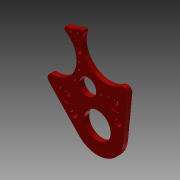
# Autodesk Inventor part: OutlineSketch1
Saved by Autodesk Inventor 2013 (Build 170138000, 138)
## iProperties
Created: 2013-06-03
Part Number: OutlineSketch1
Material: Aluminum 6061
Document SubType Name: Modeling
Designer: mvarma
Density: 2.71 g/cm^3
Mass: 149.846 g
Surface Area: 274.597 cm^2
Volume: 55.2937 cm^3
Author: mvarma
Autodesk Inventor part; units mm, degrees
ref_plane "YZ Plane" through (0, 0, 0) normal (1, 0, 0) x (0, 1, 0)
ref_plane "XZ Plane" through (0, 0, 0) normal (0, 1, 0) x (-1, 0, 0)
ref_plane "XY Plane" through (0, 0, 0) normal (0, 0, 1) x (1, 0, 0)
sketch "Sketch1" plane through (0, 0, 0) normal (0, 0, 1) x (1, 0, 0)
  line L0 (0, 0) -> (304.8, 0) construction
  line L1 (304.8, 0) -> (304.8, 50.8) construction
  line L2 (304.8, 50.8) -> (0, 50.8) construction
  line L3 (0, 50.8) -> (0, 0) construction
  circle A0 centre (152.4, 23.8125) radius 17.4625
  arc A1 (186.5267, 20.4696) -> (127.7268, 0) centre (152.4, 23.8125) ccw
  circle A2 centre (152.4, 23.8125) radius 26.035 construction
  line L4 (152.4, 23.8125) -> (139.52, 61.741) construction
  circle A3 centre (139.52, 61.741) radius 9.525 construction
  circle A4 centre (139.52, 61.741) radius 17.78 construction
  circle A5 centre (91.5619, 85.09) radius 31.75 construction
  arc A6 (133.1868, 119.4006) -> (182.1011, 83.8499) centre (163.3424, 109.4657) ccw
  circle A7 centre (109.5312, 150.0506) radius 31.75 construction
  line L5 (0, 50.8) -> (0, 53.34) construction
  line L6 (0, 53.34) -> (304.8, 53.34) construction
  line L7 (304.8, 53.34) -> (304.8, 50.8) construction
  circle A8 centre (139.52, 61.741) radius 21.59 construction
  circle A9 centre (152.4, 23.8125) radius 46.99 construction
  circle A10 centre (152.4, 23.8125) radius 50.8 construction
  arc A11 (86.3865, 79.4564) -> (92.4363, 92.6899) centre (91.5619, 85.09) ccw construction
  circle A12 centre (163.3424, 109.4657) radius 7.65 construction
  arc A13 (116.7749, 152.5104) -> (102.2875, 147.5907) centre (109.5312, 150.0506) ccw construction
  circle A14 centre (139.52, 61.741) radius 22.9 construction
  line L8 (86.3865, 79.4564) -> (124.0276, 44.8769) construction
  line L9 (170.8782, 108.1486) -> (162.078, 57.7984) construction
  line L10 (92.4363, 92.6899) -> (91.5619, 85.09) construction
  line L11 (91.5619, 85.09) -> (86.3865, 79.4564) construction
  circle A15 centre (127.6738, 96.6252) radius 3.175 construction
  circle A16 centre (127.6738, 96.6252) radius 7.9375 construction
  line L12 (92.4363, 92.6899) -> (126.7664, 88.7398) construction
  line L13 (133.1953, 90.9229) -> (158.0208, 114.9615) construction
  line L14 (158.0208, 114.9615) -> (163.3424, 109.4657) construction
  line L15 (170.8782, 108.1486) -> (163.3424, 109.4657) construction
  line L16 (139.52, 61.741) -> (127.6738, 96.6252) construction
  line L17 (91.5619, 85.09) -> (163.3424, 109.4657) construction
  line L18 (152.4, 23.8125) -> (91.5619, 85.09) construction
  line L19 (152.4, 23.8125) -> (163.3424, 109.4657) construction
  circle A17 centre (127.6738, 96.6252) radius 9.2075 construction
  circle A18 centre (127.6738, 96.6252) radius 6.1595 construction
  arc A19 (92.4363, 92.6899) -> (86.3865, 79.4564) centre (91.5619, 85.09) ccw construction
  circle A20 centre (163.3424, 109.4657) radius 25.4 construction
  circle A21 centre (109.5312, 150.0506) radius 25.4 construction
  line L20 (104.7627, 113.9656) -> (78.361, 56.2144) construction
  circle A22 centre (91.5619, 85.09) radius 25.4 construction
  line L21 (139.595, 160.2598) -> (79.4674, 139.8413) construction
  circle A23 centre (139.52, 61.741) radius 11.1125
  arc A24 (100.1373, 146.0575) -> (119.6802, 151.6232) centre (109.9088, 148.8404) ccw construction
  line L22 (109.0937, 151.2404) -> (85.4802, 141.8832) construction
  line L23 (109.9088, 148.8404) -> (85.4802, 141.8832) construction
  line L24 (109.0937, 151.2404) -> (132.7073, 160.5977) construction
  line L25 (109.9088, 148.8404) -> (134.3374, 155.7976) construction
  arc A25 (134.9211, 161.475) -> (130.4935, 159.7205) centre (132.7073, 160.5977) ccw construction
  arc A26 (132.0472, 155.1453) -> (136.6276, 156.4498) centre (134.3374, 155.7976) ccw construction
  arc A27 (132.0472, 155.1453) -> (130.4935, 159.7205) centre (85.4802, 141.8832) ccw construction
  arc A28 (136.6276, 156.4498) -> (134.9211, 161.475) centre (85.4802, 141.8832) ccw construction
  line L26 (132.7073, 160.5977) -> (134.9211, 161.475) construction
  line L27 (134.3374, 155.7976) -> (136.6276, 156.4498) construction
  arc A29 (119.6802, 151.6232) -> (118.5392, 154.9834) centre (85.4802, 141.8832) ccw construction
  arc A30 (100.1373, 146.0575) -> (99.6483, 147.4975) centre (85.4802, 141.8832) ccw construction
  line L28 (104.4015, 107.0791) -> (92.7013, 84.5343) construction
  line L29 (81.0012, 61.9895) -> (90.3961, 85.5882) construction
  arc A31 (100.6718, 111.3992) -> (98.9102, 106.9744) centre (99.791, 109.1868) ccw construction
  arc A32 (103.3046, 104.9655) -> (105.4983, 109.1926) centre (104.4015, 107.0791) ccw construction
  arc A33 (103.3046, 104.9655) -> (98.9102, 106.9744) centre (81.0012, 61.9895) ccw construction
  line L30 (99.791, 109.1868) -> (100.6718, 111.3992) construction
  line L31 (104.4015, 107.0791) -> (105.4983, 109.1926) construction
  arc A34 (105.4983, 109.1926) -> (100.6718, 111.3992) centre (81.0012, 61.9895) ccw construction
  arc A35 (118.5392, 154.9834) -> (99.6483, 147.4975) centre (109.0937, 151.2404) ccw construction
  arc A36 (88.0213, 75.5164) -> (97.3814, 93.5522) centre (92.7013, 84.5343) ccw construction
  line L32 (90.3961, 85.5882) -> (99.791, 109.1868) construction
  line L33 (92.7013, 84.5343) -> (81.0012, 61.9895) construction
  arc A37 (88.0213, 75.5164) -> (86.6381, 76.1487) centre (81.0012, 61.9895) ccw construction
  arc A38 (97.3814, 93.5522) -> (94.1541, 95.0276) centre (81.0012, 61.9895) ccw construction
  arc A39 (94.1541, 95.0276) -> (86.6381, 76.1487) centre (90.3961, 85.5882) ccw construction
  line L34 (163.3424, 109.4657) -> (140.8985, 121.3583) construction
  line L35 (163.3424, 109.4657) -> (185.7862, 97.5731) construction
  circle A40 centre (139.52, 61.741) radius 22.9 construction
  arc A41 (102.2875, 147.5907) -> (116.7749, 152.5104) centre (109.5312, 150.0506) ccw construction
  arc A42 (102.2875, 147.5907) -> (102.6226, 146.7653) centre (109.5312, 150.0506) ccw construction
  circle A43 centre (90.3961, 85.5882) radius 31.75
  arc A44 (107.3265, 112.7153) -> (92.5282, 52.7848) centre (92.7013, 84.5343) ccw
  line L36 (100.6718, 111.3992) -> (102.1397, 115.0865) construction
  line L37 (105.4983, 109.1926) -> (107.3265, 112.7153) construction
  arc A45 (107.3265, 112.7153) -> (102.1397, 115.0865) centre (81.0012, 61.9895) ccw
  circle A46 centre (109.0937, 151.2404) radius 31.75
  arc A47 (120.148, 118.7867) -> (128.3292, 122.9801) centre (109.9088, 148.8404) ccw
  line L38 (134.9211, 161.475) -> (138.6107, 162.9371) construction
  line L39 (136.6276, 156.4498) -> (140.4445, 157.5369) construction
  arc A48 (140.4445, 157.5369) -> (138.6107, 162.9371) centre (85.4802, 141.8832) ccw
  line L40 (91.5619, 85.09) -> (109.5312, 150.0506) construction
  line L41 (109.5312, 150.0506) -> (163.3424, 109.4657) construction
  line L42 (139.52, 61.741) -> (109.5312, 150.0506) construction
  circle A49 centre (139.52, 61.741) radius 17.4625
  line L43 (139.52, 61.741) -> (122.0575, 61.741) construction
  line L44 (139.52, 61.741) -> (156.9825, 61.741) construction
  line L45 (139.52, 61.741) -> (156.9825, 61.741) construction
  circle A50 centre (139.52, 61.741) radius 26.71 construction
  circle A51 centre (111.304, 39.007) radius 9.525 construction
  circle A52 centre (175.745, 60.8903) radius 9.525 construction
  line L46 (0, 3.81) -> (304.8, 3.81) construction
  arc A53 (86.5066, 75.4886) -> (95.7233, 93.5981) centre (91.1149, 84.5434) ccw
  arc A54 (92.4843, 95.0479) -> (85.1185, 76.1099) centre (88.8014, 85.5789) ccw
  arc A55 (95.7233, 93.5981) -> (92.4843, 95.0479) centre (79.5941, 61.9064) ccw
  circle A56 centre (120.9278, 20.7284) radius 5.588
  circle A57 centre (179.6201, 39.9084) radius 5.588
  line L47 (152.4, 23.8125) -> (304.8, 25.4) construction
  line L48 (179.6201, 39.9084) -> (152.4, 23.8125) construction
  line L49 (152.4, 23.8125) -> (120.9278, 20.7284) construction
  line L50 (67.3436, 63.7559) -> (87.8831, 42.0684)
  line L51 (186.5267, 20.4696) -> (192.1727, 78.1076)
  arc A58 (109.8133, 111.2783) -> (111.3776, 117.1243) centre (111.5245, 113.9527) ccw
  arc A59 (128.3292, 122.9801) -> (133.1868, 119.4006) centre (130.1712, 120.3941) ccw
  arc A60 (111.3776, 117.1243) -> (120.148, 118.7867) centre (109.9088, 148.8404) ccw
  arc A61 (128.3292, 122.9801) -> (111.3776, 117.1243) centre (109.9088, 148.8404) ccw
  arc A62 (137.9937, 128.5839) -> (133.1868, 119.4006) centre (163.3424, 109.4657) ccw
  arc A63 (109.8133, 111.2783) -> (107.3265, 112.7153) centre (92.7013, 84.5343) ccw
  arc A64 (92.5282, 52.7848) -> (87.8831, 42.0684) centre (92.4936, 46.4349) ccw
  arc A65 (182.1011, 83.8499) -> (192.1727, 78.1076) centre (185.8529, 78.7267) ccw
  arc A66 (192.1727, 78.1076) -> (182.1011, 83.8499) centre (185.8529, 78.7267) ccw
  arc A67 (97.1053, 50.8) -> (92.5282, 52.7848) centre (92.4936, 46.4349) ccw
  arc A68 (87.8831, 42.0684) -> (97.1053, 50.8) centre (92.4936, 46.4349) ccw
  line L52 (87.8831, 42.0684) -> (127.5033, 0.2337)
  line L53 (192.1727, 78.1076) -> (194.9412, 106.3704)
  arc A69 (182.1011, 83.8499) -> (137.9937, 128.5839) centre (163.3424, 109.4657) ccw
  arc A70 (180.2515, 3.81) -> (186.5267, 20.4696) centre (152.4, 23.8125) ccw
  arc A71 (127.7268, 0) -> (180.2515, 3.81) centre (152.4, 23.8125) ccw
  arc A72 (92.5282, 52.7848) -> (109.8133, 111.2783) centre (92.7013, 84.5343) ccw
  arc A73 (133.1868, 119.4006) -> (128.3292, 122.9801) centre (130.1712, 120.3941) ccw
  arc A74 (111.3776, 117.1243) -> (109.8133, 111.2783) centre (111.5245, 113.9527) ccw
  point P0 (133.5823, 158.218)
  point P1 (102.1225, 108.1905)
  dimension "d122" = 63.5
  dimension "d1" = 50.8
  dimension "d2" = 34.925
  dimension "d3" = 23.8125
  dimension "d4" = 152.4
  dimension "d7" = 68.58
  dimension "d8" = 52.07
  dimension "d9" = 19.05
  dimension "d10" = 35.56
  dimension "d11" = 40.0558
  dimension "d12" = 63.5
  dimension "d13" = 63.5
  dimension "d14" = 63.5
  dimension "d15" = 2.54
  dimension "d16" = 304.8
  dimension "d17" = 43.18
  dimension "d18" = 93.98
  dimension "d19" = 101.6
  dimension "d21" = 15.3
  dimension "d22" = 15.3
  dimension "d29" = 45.8
  dimension "d30" = 143.991
  dimension "d31" = 6.35
  dimension "d32" = 15.875
  dimension "d33" = 143.991
  dimension "d35" = 18.415
  dimension "d37" = 12.319
  dimension "d40" = 50.8
  dimension "d41" = 50.8
  dimension "d42" = 18.004
  dimension "d43" = 18.004
  dimension "d44" = 50.8
  dimension "d57" = 22.225
  dimension "d67" = 25.4
  dimension "d68" = 25.4
  dimension "d69" = 2.86
  dimension "d70" = 25.4
  dimension "d71" = 25.4
  dimension "d72" = 4.7625
  dimension "d75" = 2.86
  dimension "d80" = 4.7625
  dimension "d82" = 4.7625
  dimension "d83" = 50.8
  dimension "d84" = 50.8
  dimension "d85" = 10.16
  dimension "d97" = 48.4188
  dimension "d99" = 20.32
  dimension "d101" = 25.4
  dimension "d102" = 25.4
  dimension "d103" = 10.16
  dimension "d105" = 18.004
  dimension "d106" = 18.004
  dimension "d107" = 45.8
  dimension "d109" = 7.65
  dimension "d114" = 63.5
  dimension "d115" = 63.5
  dimension "d116" = 57.15
  dimension "d123" = 63.5
  dimension "d128" = 93.2626
  dimension "d129" = 34.925
  dimension "d130" = 0
  dimension "d138" = 53.42
  dimension "d139" = 19.05
  dimension "d140" = 19.05
  dimension "d154" = 3.81
  constraints: 124 point on circle, 108 end point, 74 centre point, 48 coincident, 43 tangent, 23 point on line, 15 collinear, 8 perpendicular, 3 midpoint, 3 parallel, 2 equal radius, 2 horizontal, 1 equal length, 12 other
  measures "d1" distance of L1.end L0.end
  measures "d2" diameter of A0
  measures "d3" distance from line of L0 A0.centre
  measures "d4" distance from line of L3 A0.centre
  measures "d7" diameter of A1
  measures "d8" diameter of A2
  measures "d9" diameter of A3
  measures "d10" diameter of A4
  measures "d11" distance of L4.start L4.end
  measures "d12" diameter of A5
  measures "d13" diameter of A6
  measures "d14" diameter of A7
  measures "d15" distance of L2.end L5.end
  measures "d16" distance of L0.end L0.start
  measures "d17" diameter of A8
  measures "d18" diameter of A9
  measures "d19" diameter of A10
  measures "d21" diameter of A11
  measures "d22" diameter of A12
  measures "d29" diameter of A14
  measures "d30" angle of L11 L10
  measures "d31" diameter of A15
  measures "d32" diameter of A16
  measures "d33" angle of L15 L14
  measures "d35" diameter of A17
  measures "d37" diameter of A18
  measures "d40" diameter of A20
  measures "d41" diameter of A21
  measures "d42" angle of L10 L20
  measures "d43" angle of L11 L20
  measures "d44" diameter of A22
  measures "d57" diameter of A23
  measures "d67" distance of L22.start L22.end
  measures "d68" distance of L23.start L22.end
  measures "d69" angle of L21 L22
  measures "d70" distance of L22.start L24.end
  measures "d71" distance of L23.start L25.end
  measures "d72" diameter of A25
  measures "d75" angle of L20 L28
  measures "d80" diameter of A31
  measures "d82" diameter of A32
  measures "d83" distance of L29.start L32.end
  measures "d84" distance of L28.start L29.start
  measures "d85" radius of A24
  measures "d97" radius of A33
  measures "d99" diameter of A36
  measures "d101" distance of L29.start L29.end
  measures "d102" distance of L28.end L29.start
  measures "d103" radius of A39
  measures "d105" angle of L34 L14
  measures "d106" angle of L35 L15
  measures "d107" diameter of A40
  measures "d109" radius of A13
  measures "d114" diameter of A43
  measures "d115" diameter of A44
  measures "d116" radius of A45
  measures "d123" diameter of A47
  measures "d128" distance of L42.start L40.end
  measures "d129" diameter of A49
  measures "d130" distance between parallel lines of L45 L44
  measures "d138" diameter of A50
  measures "d139" diameter of A51
  measures "d140" diameter of A52
  measures "d154" distance between parallel lines of L0 L46
extrude "Plates" add sketch "Sketch1" along normal blind 6.35 contours A0 | A1 A56 A49 A57 A70 A71 | L52 A68 A67 A72 A58 A60 A47 A59 A6 A65 L51 A1 A57 A49 A56 | A56 A1 | A1 A56 | A64 A67 A68 | A49 A1 A23 | A1 A23 A49 | A74 A58 | A57 A1 | A1 A57 | A65 A66 | A23 A1 | A1 A23 | A59 A73
extrude "Bearing Cuts" cut sketch "Sketch1" along normal blind 25.4 contours A0 | A23 A1 | A1 A23
hole "Encoder Mounting Holes" at (122.0575, 61.741, 0) at (156.9825, 61.741, 0) direction (0, 0, 1) diameter 2.6416 end through all thread size "6-32 UNC" class "2B" standard "ANSI Unified Screw Threads"
hole "10-32 Pem Nut Holes" at (81.0012, 61.9895, 0) at (85.4802, 141.8832, 0) at (100.6718, 111.3992, 0) at (105.4983, 109.1926, 0) at (102.1225, 108.1905, 0) at (127.6738, 96.6252, 0) at (111.304, 39.007, 0) at (175.745, 60.8903, 0) direction (0, 0, 1) diameter 6.35 end through all
hole "1/4-20 Pem Nut Holes" at (185.7862, 97.5731, 0) at (140.8985, 121.3583, 0) at (120.9278, 20.7284, 0) at (179.6201, 39.9084, 0) at (133.5823, 158.218, 0) direction (0, 0, 1) diameter 8.7376 end through all
sketch "Sketch5" plane through (0, 0, 0) normal (0, 0, -1) x (-1, 0, 0)
  line L0 (-124.4513, 85.236) -> (-124.4513, 75.711)
  line L1 (-124.4513, 85.236) -> (-127.6263, 85.236)
  line L2 (-127.6263, 85.236) -> (-127.6263, 75.711)
  line L3 (-127.6263, 75.711) -> (-124.4513, 75.711)
  line L4 (-139.52, 61.741) -> (-109.9088, 148.8404) construction
  line L5 (-124.6374, 120.313) -> (-115.6193, 117.2471) construction
  line L6 (-124.6374, 120.313) -> (-125.6594, 117.307) construction
  line L7 (-125.6594, 117.307) -> (-116.6413, 114.2411) construction
  line L8 (-116.6413, 114.2411) -> (-115.6193, 117.2471) construction
  circle A0 centre (-139.52, 61.741) radius 11.1125 projected
  arc A1 (-128.3292, 122.9801) -> (-111.3776, 117.1243) centre (-109.9088, 148.8404) ccw projected
  arc A2 (-109.8133, 111.2783) -> (-92.5282, 52.7848) centre (-92.7013, 84.5343) ccw projected
  dimension "d196" = 9.525
  dimension "d198" = 3.175
  dimension "d201" = 13.97
  dimension "d209" = 9.525
  dimension "d210" = 3.175
  constraints: 18 end point, 6 coincident, 5 perpendicular, 2 parallel, 2 tangent, 1 symmetric about line, 1 vertical
  measures "d196" distance of L0.start L0.end
  measures "d198" distance of L0.start L1.end
  measures "d201" vertical distance of L4.start point (-127.626, 75.711)
  measures "d209" distance of L5.start L5.end
  measures "d210" distance of L5.start L6.end
hole "Cim Adjustment Block Holes" at (127.6263, 85.236, 0) at (127.6263, 75.711, 0) at (125.6594, 117.307, 0) at (116.6413, 114.2411, 0) direction (0, 0, 1) diameter 2.6416 end through all thread size "6-32 UNC" class "2B" standard "ANSI Unified Screw Threads"
sketch "Sketch8" plane through (0, 0, 6.35) normal (0, 0, 1) x (1, 0, 0)
  circle A0 centre (111.304, 39.007) radius 3.175 projected
  circle A1 centre (175.745, 60.8903) radius 3.175 projected
  circle A2 centre (111.304, 39.007) radius 9.525
  circle A3 centre (175.745, 60.8903) radius 9.525
  point P0 (0, 0)
  dimension "d235" = 19.05
  dimension "d236" = 19.05
  constraints: 2 centre point, 2 coincident
  measures "d235" diameter of A2
  measures "d236" diameter of A3
extrude "Extrusion5" cut sketch "Sketch8" against normal blind 1.1906
sketch "Sketch9" plane through (0, 0, 0) normal (0, 0, -1) x (-1, 0, 0)
  circle A0 centre (-111.304, 39.007) radius 3.175 projected
  circle A1 centre (-175.745, 60.8903) radius 3.175 projected
  circle A2 centre (-175.745, 60.8903) radius 9.525 projected
  circle A3 centre (-125.6594, 117.307) radius 1.3208 projected
  circle A4 centre (-127.6263, 85.236) radius 1.3208 projected
  circle A5 centre (-127.6263, 75.711) radius 1.3208 projected
  circle A6 centre (-116.6413, 114.2411) radius 1.3208 projected
  circle A7 centre (-179.6201, 39.9084) radius 4.3688 projected
  circle A8 centre (-120.9278, 20.7284) radius 4.3688 projected
  circle A9 centre (-111.304, 39.007) radius 3.175 projected
  circle A10 centre (-127.6738, 96.6252) radius 3.175 projected
  circle A11 centre (-175.745, 60.8903) radius 3.175 projected
  circle A12 centre (-122.0575, 61.741) radius 1.3208 projected
  circle A13 centre (-156.9825, 61.741) radius 1.3208 projected
  circle A14 centre (-152.4, 23.8125) radius 17.4625 projected
  circle A15 centre (-139.52, 61.741) radius 11.1125 projected
  arc A16 (-182.1011, 83.8499) -> (-192.1727, 78.1076) centre (-185.8529, 78.7267) ccw projected
  line L0 (-186.5267, 20.4696) -> (-192.1727, 78.1076) projected
  arc A17 (-186.5267, 20.4696) -> (-127.5033, 0.2337) centre (-152.4, 23.8125) ccw projected
  line L1 (-87.8831, 42.0684) -> (-127.5033, 0.2337) projected
  arc A18 (-87.8831, 42.0684) -> (-92.5282, 52.7848) centre (-92.4936, 46.4349) ccw projected
  arc A19 (-109.8133, 111.2783) -> (-92.5282, 52.7848) centre (-92.7013, 84.5343) ccw projected
  arc A20 (-109.8133, 111.2783) -> (-111.3776, 117.1243) centre (-111.5245, 113.9527) ccw projected
  arc A21 (-128.3292, 122.9801) -> (-111.3776, 117.1243) centre (-109.9088, 148.8404) ccw projected
  arc A22 (-128.3292, 122.9801) -> (-133.1868, 119.4006) centre (-130.1712, 120.3941) ccw projected
  arc A23 (-182.1011, 83.8499) -> (-133.1868, 119.4006) centre (-163.3424, 109.4657) ccw projected
  circle A24 centre (-111.304, 39.007) radius 9.525 projected
  point P0 (0, 0)
extrude "Extrusion6" cut sketch "Sketch9" against normal blind 1.1906 contours A2 | A24
equation "\"d9\" = Gear15tPD"
equation "\"d10\" = Gear28tPD"
equation "\"d11\" = 0.5 * Gear48tPD + 0.5 * Gear15tPD + MeshingClearance"
equation "\"d12\" = CimOD"
equation "\"d13\" = CimOD"
equation "\"d14\" = CimOD"
equation "\"d17\" = Gear28tPD + ClearanceDiameter"
equation "\"d18\" = WheelOD"
equation "\"d19\" = WheelClearance"
equation "\"Pulley48tPD\" = 45.8"
equation "\"Pulley19tPD\" = 18.2"
equation "\"Pulley16tPD\" = 15.3"
equation "\"Gear15tPD\" = 19.05"
equation "\"Gear35tPD\" = 44.45"
equation "\"Gear48tPD\" = 60.96"
equation "\"Gear28tPD\" = 35.56"
equation "\"BearingLargeOD\" = 28.575"
equation "\"BearingSmallOD\" = 22.225"
equation "\"MeshingClearance\" = 0.0508"
equation "\"CimOD\" = 63.5"
equation "\"WheelOD\" = 93.98"
equation "\"ClearanceDiameter\" = 7.62"
equation "\"WheelClearance\" = 101.6"
equation "\"TensioningBearingID\" = 6.35"
equation "\"TensioningBearingOD\" = 15.875"
equation "\"SpingClipClearance\" = 8.89"
equation "\"Pi\" = 79.79645"
equation "\"Pulley56tPD\" = 53.5"
equation "\"BearingXLargeOD\" = 34.925"
body "Solid3"
